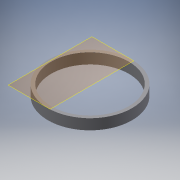
# Autodesk Inventor part: 27_Lens_Ring
Saved by Autodesk Inventor 2016 (Build 200138000, 138)
## iProperties
Created: 2016-12-10
Part Number: 27_Lens_Ring
Material: Generisch
Document SubType Name: Modeling
Designer: Bene
Density: 1 g/cm^3
Appearance: Vorgabe
Author: Bene
Autodesk Inventor part; units mm, degrees
ref_plane "YZ Plane" through (0, 0, 0) normal (1, 0, 0) x (0, 1, 0)
ref_plane "XZ Plane" through (0, 0, 0) normal (0, 1, 0) x (-1, 0, 0)
ref_plane "XY Plane" through (0, 0, 0) normal (0, 0, 1) x (1, 0, 0)
ref_plane "Arbeitsebene1" through (0, 0, 0) normal (0, 0, 1) x (1, 0, 0)
sketch "Skizze1" plane through (0, 0, 0) normal (0, 0, 1) x (1, 0, 0)
  arc A0 (0, -13.419) -> (0, 13.419) centre (0, 0) ccw projected
  line L0 (0, 14.5) -> (0, 12.5) projected
  arc A1 (0, -12.5) -> (0, 12.5) centre (0, 0) ccw projected
  line L1 (0, -12.5) -> (0, -14.5) projected
  arc A2 (0, -14.5) -> (0, 14.5) centre (0, 0) ccw projected
  circle A3 centre (0, 0) radius 14.75
  circle A4 centre (0, 0) radius 16
  circle A5 centre (0, 0) radius 13.419 projected
  circle A6 centre (0, 0) radius 12.5 projected
  circle A7 centre (0, 0) radius 14.5 projected
  dimension "d0" = 29.5
  dimension "d1" = 32
  constraints: 2 centre point, 1 coincident
  measures "d0" diameter of A3
  measures "d1" diameter of A4
extrude "Extrusion1" add sketch "Skizze1" against normal blind 4 contours A4
